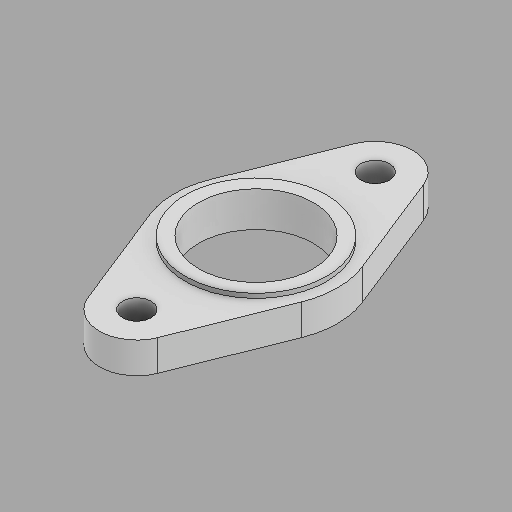
# Autodesk Inventor part: 00.32.011 "Flange"
Saved by Autodesk Inventor 2025.2 (Build 292293000, 293)
## iProperties
Created: 2024-12-15
Part Number: 00.32.011 "Flange"
Material: Generic
Document SubType Name: Modeling
Designer: Anna
Density: 1 g/cm^3
Appearance: Default
Author: Anna
Autodesk Inventor part; units mm, degrees
ref_plane "YZ Plane" through (0, 0, 0) normal (1, 0, 0) x (0, 1, 0)
ref_plane "XZ Plane" through (0, 0, 0) normal (0, 1, 0) x (-1, 0, 0)
ref_plane "XY Plane" through (0, 0, 0) normal (0, 0, 1) x (1, 0, 0)
sketch "Sketch1" plane through (0, 0, 0) normal (0, 1, 0) x (-1, 0, 0)
  arc A0 (17.4776, 61.9438) -> (-14.1045, 61.9438) centre (1.6865, 55.6475) ccw
  arc A1 (-14.1045, -58.6488) -> (17.4776, -58.6488) centre (1.6865, -52.3525) ccw
  line L0 (36.0552, 15.3512) -> (17.4776, 61.9438)
  line L1 (-14.1045, 61.9438) -> (-32.6822, 15.3512)
  line L2 (-32.6822, -12.0562) -> (-14.1045, -58.6488)
  line L3 (17.4776, -58.6488) -> (36.0552, -12.0562)
  arc A2 (-32.6822, 15.3512) -> (-32.6822, -12.0562) centre (1.6865, 1.6475) ccw
  arc A3 (36.0552, -12.0562) -> (36.0552, 15.3512) centre (1.6865, 1.6475) ccw
  circle A4 centre (1.6865, 55.6475) radius 6.5
  circle A5 centre (1.6865, -52.3525) radius 6.5
  circle A6 centre (1.6865, 1.6475) radius 26
  dimension "d11" = 13
  dimension "d12" = 13
  dimension "d13" = 52
  constraints: 8 end point, 8 point on circle, 8 tangent, 7 centre point, 3 coincident
  measures "d11" diameter of A4
  measures "d12" diameter of A5
  measures "d13" diameter of A6
extrude "Extrusion1" add sketch "Sketch1" along normal blind 14
sketch "Sketch2" plane through (0, 14, 0) normal (0, 1, 0) x (1, 0, 0)
  circle A0 centre (-1.6865, -1.6475) radius 26 projected
  circle A1 centre (-1.6865, -1.6475) radius 32
  point P0 (0, 0)
  dimension "d16" = 64
  constraints: 1 centre point, 1 coincident
  measures "d16" diameter of A1
extrude "Extrusion2" add sketch "Sketch2" along normal blind 2
body "Solid1"
